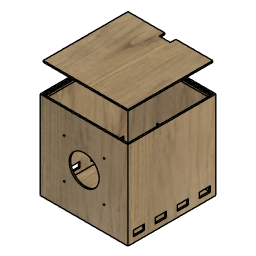
NoteBlockMaestro (Autodesk Fusion 360 design; units mm, degrees)
part number: 2025-07-01-10-41-04-519
Autodesk Fusion 360 part; units mm, degrees
sketch "Sketch1" plane through (0, 0, 0) normal (0, 0, 1) x (1, 0, 0)
  line L0 (0, 0) -> (152, 0)
  line L1 (152, 0) -> (152, -152)
  line L2 (152, -152) -> (0, -152)
  line L3 (0, -152) -> (0, 0)
  dimension "d1" = 152
  dimension "d2" = 152
  constraint horizontal L0
  constraint vertical L1
  constraint horizontal L2
  constraint vertical L3
  constraint coincident L0.start L3.end
  measures "d1" distance of L0.start L0.end
  measures "d2" distance of L0.start L2.end
extrude "Extrude1" add sketch "Sketch1" along normal blind 152 makes body 1
move_body "Move1" bodies 1 to x (1, 0, 0) y (0, 1, 0) z (0, 0, 1) at (76, 0, 0)
move_body "Move2" bodies 1 to x (1, 0, 0) y (0, 1, 0) z (0, 0, 1) at (-152, 0, 0)
move_body "Move3" bodies 1 to x (1, 0, 0) y (0, 1, 0) z (0, 0, 1) at (0, -76, 0)
move_body "Move4" bodies 1 to x (1, 0, 0) y (0, 1, 0) z (0, 0, 1) at (0, 152, 0)
shell "Shell1" thickness 2.5 removed faces 1 at (-25.3333, 25.3333, 152) on bodies 1
sketch "Sketch2" plane through (0, 0, 152) normal (0, 0, 1) x (-1, 0, 0)
  line L0 (73.5, 73.5) -> (73.5, -73.5)
  line L1 (73.5, -73.5) -> (-73.5, -73.5)
  line L2 (-73.5, -73.5) -> (-73.5, 73.5)
  line L3 (-73.5, 73.5) -> (73.5, 73.5)
  line L4 (76, 76) -> (-76, 76)
  line L5 (-76, 76) -> (-76, -76)
  line L6 (-76, -76) -> (76, -76)
  line L7 (76, -76) -> (76, 76)
  line L8 (76, -76) -> (-76, -76)
  line L9 (-76, -76) -> (-76, 76)
  line L10 (-76, 76) -> (76, 76)
  line L11 (76, 76) -> (76, -76)
  constraint horizontal L8
  constraint vertical L9
  constraint horizontal L10
  constraint vertical L11
  constraint coincident L4.end L5.start
  constraint coincident L6.end L7.start
extrude "Extrude2" add sketch "Sketch2" along normal blind 2.5 separate body contours L0 L1 L2 L3 makes body 2
move_body "Move5" bodies 2 to x (1, 0, 0) y (0, 1, 0) z (0, 0, 1) at (0, 0, 100)
ref_plane "WorkPlane1" through (0, 0, 149.5) normal (0, 0, 1) x (1, 0, 0)
sketch "Sketch3" plane through (0, 0, 149.5) normal (0, 0, 1) x (1, 0, 0)
  line L0 (73.5, 73.5) -> (-73.5, 73.5)
  line L1 (-73.5, 73.5) -> (-73.5, -73.5)
  line L2 (-73.5, -73.5) -> (73.5, -73.5)
  line L3 (73.5, -73.5) -> (73.5, 73.5)
  line L4 (-72.5, -72.5) -> (72.5, -72.5)
  line L5 (72.5, -72.5) -> (72.5, 72.5)
  line L6 (72.5, 72.5) -> (-72.5, 72.5)
  line L7 (-72.5, 72.5) -> (-72.5, -72.5)
  point P0 (-73.5, 73.5)
  point P1 (73.5, 73.5)
  point P2 (-73.5, -73.5)
  point P3 (73.5, -73.5)
  dimension "d9" = -1
  constraint horizontal L0
  constraint vertical L1
  constraint horizontal L2
  constraint vertical L3
  constraint coincident P2 L1.end
  constraint coincident P1 L0.start
extrude "Extrude3" add sketch "Sketch3" against normal blind 2 bodies 1
extrude "Extrude4" add 1 faces at (-72.5, 24.1667, 148.8333) along direction (1, 0, 0) blind 1 on bodies 1 bodies 1
extrude "Extrude5" add 1 faces at (24.5, 72.5, 148.8333) along direction (0, -1, 0) blind 1 on bodies 1 bodies 1
extrude "Extrude6" add 1 faces at (72.5, -24.5, 148.8333) along direction (-1, 0, 0) blind 1 on bodies 1 bodies 1
extrude "Extrude7" add 1 faces at (-23.8333, -72.5, 148.1667) along direction (0, 1, 0) blind 1 on bodies 1 bodies 1
extrude "Extrude8" add 1 faces at (-73.5, -24.5, 252.8333) along direction (-1, 0, 0) blind 0.1 on bodies 2 bodies 2
extrude "Extrude9" cut 1 faces at (-73.6, -24.5, 252.8333) along direction (1, 0, 0) blind 0.2 on bodies 2 bodies 2
extrude "Extrude10" cut 1 faces at (24.5333, -73.5, 252.8333) along direction (0, 1, 0) blind 0.2 on bodies 2 bodies 2
extrude "Extrude11" cut 1 faces at (73.5, 24.5667, 252.8333) along direction (-1, 0, 0) blind 0.2 on bodies 2 bodies 2
extrude "Extrude12" cut 1 faces at (-24.5, 73.5, 253.6667) along direction (0, -1, 0) blind 0.2 on bodies 2 bodies 2
move_body "Move6" bodies 2 to x (1, 0, 0) y (0, 1, 0) z (0, 0, 1) at (0, 0, -60)
sketch "Sketch4" plane through (0, 0, 194.5) normal (0, 0, 1) x (-1, 0, 0)
  line L0 (-73.3, -73.3) -> (73.4, -73.3)
  line L1 (73.4, -73.3) -> (73.4, 73.3)
  line L2 (73.4, 73.3) -> (-73.3, 73.3)
  line L3 (-73.3, 73.3) -> (-73.3, -73.3)
  line L4 (0.05, -73.3) -> (9.55, -73.3)
  line L5 (0.05, -73.3) -> (-9.45, -73.3)
  line L6 (-9.45, -73.3) -> (-9.45, -63.8)
  line L7 (-9.45, -63.8) -> (0.05, -63.8)
  line L8 (0.05, -63.8) -> (9.55, -63.8)
  line L9 (9.55, -63.8) -> (9.55, -73.3)
  dimension "d30" = 9.5
  dimension "d31" = 9.5
  dimension "d32" = 9.5
  dimension "d33" = 9.5
  dimension "d34" = 9.5
  dimension "d35" = 9.5
  constraint midpoint L0 L4.start
  constraint parallel L0 L4
  constraint parallel L0 L5
  constraint perpendicular L5 L6
  constraint perpendicular L6 L7
  constraint perpendicular L6 L8
  constraint perpendicular L4 L9
  measures "d30" distance of L4.start L4.end
  measures "d31" distance of L4.start L5.end
  measures "d32" distance of L5.end L6.end
  measures "d33" distance of L6.end L7.end
  measures "d34" distance of L7.end L8.end
  measures "d35" distance of L8.end L4.end
extrude "Extrude13" cut sketch "Sketch4" against normal blind 2.5 contours L0 L4 L5 L6 L7 L8 L9 bodies 2
move_body "Move7" bodies 2 to x (1, 0, 0) y (0, 1, 0) z (0, 0, 1) at (0, 0, -42.5)
sketch "Sketch5" plane through (0, 0, 149.5) normal (0, 0, 1) x (-1, 0, 0)
  line L0 (71.5, 71.5) -> (71.5, -71.5)
  line L1 (71.5, -71.5) -> (-71.5, -71.5)
  line L2 (-71.5, -71.5) -> (-71.5, 71.5)
  line L3 (-71.5, 71.5) -> (71.5, 71.5)
  line L4 (-73.5, 73.5) -> (-73.5, -73.5)
  line L5 (-73.5, -73.5) -> (73.5, -73.5)
  line L6 (73.5, -73.5) -> (73.5, 73.5)
  line L7 (73.5, 73.5) -> (-73.5, 73.5)
  line L8 (9.55, -73.5) -> (-9.4425, -73.5)
  line L9 (-9.4425, -73.5) -> (-9.4425, -71.5)
  line L10 (-9.4425, -71.5) -> (9.55, -71.5)
  line L11 (9.55, -71.5) -> (9.55, -73.5)
  constraint horizontal L8
  constraint vertical L9
  constraint horizontal L10
  constraint vertical L11
  constraint coincident L1 L9.end
  constraint coincident L5 L8.start
extrude "Extrude14" cut sketch "Sketch5" against normal blind 2 contours L1 L5 L8 L9 L10 L11 bodies 1
move_body "Move8" bodies 2 to x (1, 0, 0) y (0, 1, 0) z (0, 0, 1) at (0, 0, 50)
extrude "Extrude15" add 1 faces at (71.5, -23.8333, 148.1667) along direction (-1, 0, 0) blind 0.5 on bodies 1 bodies 1
extrude "Extrude16" add 1 faces at (50.4808, 71.5, 148.8333) along direction (0, -1, 0) blind 0.5 on bodies 1 bodies 1
extrude "Extrude17" add 1 faces at (-71.5, 23.8333, 148.1667) along direction (1, 0, 0) blind 0.5 on bodies 1 bodies 1
extrude "Extrude18" add 1 faces at (-23.6667, -71.5, 148.8333) along direction (0, 1, 0) blind 0.5 on bodies 1 bodies 1
extrude "Extrude19" add 1 faces at (-23.6667, -72.6667, 147.5) along direction (0, 0, -1) blind 0.5 on bodies 1 bodies 1
extrude "Extrude20" add 1 faces at (-23.6667, -72.6667, 147) along direction (0, 0, -1) blind 1 on bodies 1 bodies 1
scale "Scale1" factor 1.157895 about (71, -71, 146) bodies 1 2
move_face "MoveFace1" by (70, 0, 0) 1 faces at (-40.5439, 99.2105, 94.2807) on bodies 1
move_body "Move9" bodies 1 2 to x (1, 0, 0) y (0, 1, 0) z (0, 0, 1) at (11, 0, 0)
move_body "Move10" bodies 1 2 to x (1, 0, 0) y (0, 1, 0) z (0, 0, 1) at (0, -11, 0)
move_body "Move11" bodies 1 2 to x (1, 0, 0) y (0, 1, 0) z (0, 0, 1) at (0, 0, 23)
sketch "Sketch8" plane through (0, 88.2105, 0) normal (0, 1, 0) x (-1, 0, 0)
  line L0 (-87.7895, -0.0526) -> (88.2105, -0.0526)
  line L1 (88.2105, -0.0526) -> (88.2105, 175.9474)
  line L2 (88.2105, 175.9474) -> (-87.7895, 175.9474)
  line L3 (-87.7895, 175.9474) -> (-87.7895, -0.0526)
  line L4 (0, 25) -> (27.5, 25)
  line L5 (0, 25) -> (-27.5, 25)
  line L6 (-27.5, 25) -> (-27.5, 69)
  line L7 (-27.5, 69) -> (27.5, 69)
  line L8 (27.5, 69) -> (27.5, 25)
  dimension "d54" = 27.5
  dimension "d55" = 27.5
  dimension "d56" = 44
  dimension "d57" = 55
  constraint horizontal L4
  constraint horizontal L5
  constraint perpendicular L5 L6
  constraint perpendicular L6 L7
  measures "d54" distance of L4.start L4.end
  measures "d55" distance of L4.start L5.end
  measures "d56" distance of L5.end L6.end
  measures "d57" distance of L6.end L7.end
extrude "Extrude21" cut sketch "Sketch8" against normal blind 3 contours L4 L5 L6 L7 L8 bodies 1
sketch "Sketch9" plane through (-88.2105, 0, 0) normal (-1, 0, 0) x (0, -1, 0)
  line L0 (-88.2105, -0.0526) -> (87.7895, -0.0526)
  line L1 (87.7895, -0.0526) -> (87.7895, 175.9474)
  line L2 (87.7895, 175.9474) -> (-88.2105, 175.9474)
  line L3 (-88.2105, 175.9474) -> (-88.2105, -0.0526)
  line L4 (11, 11) -> (11, 22)
  line L5 (11, 22) -> (33, 22)
  line L6 (33, 22) -> (33, 11)
  line L7 (33, 11) -> (11, 11)
  line L8 (55, 22) -> (77, 22)
  line L9 (77, 22) -> (77, 11)
  line L10 (77, 11) -> (55, 11)
  line L11 (55, 11) -> (55, 22)
  line L12 (-11, 11) -> (-33, 11)
  line L13 (-33, 11) -> (-33, 22)
  line L14 (-33, 22) -> (-11, 22)
  line L15 (-11, 22) -> (-11, 11)
  line L16 (-55, 11) -> (-77, 11)
  line L17 (-77, 11) -> (-77, 22)
  line L18 (-77, 22) -> (-55, 22)
  line L19 (-55, 22) -> (-55, 11)
  dimension "d61" = 11
  dimension "d62" = 22
  dimension "d64" = 22
  dimension "d65" = 11
  dimension "d67" = 22
  dimension "d68" = 11
  constraint perpendicular L4 L5
  constraint perpendicular L5 L6
  constraint perpendicular L4 L7
  constraint perpendicular L0 L9
  constraint perpendicular L6 L10
  constraint perpendicular L12 L13
  constraint perpendicular L13 L14
  constraint perpendicular L13 L16
  constraint perpendicular L13 L18
  constraint perpendicular L16 L19
  measures "d61" distance of L4.start L4.end
  measures "d62" distance of L4.end L5.end
  measures "d64" distance of L8.start L8.end
  measures "d65" distance of L8.end L9.end
  measures "d67" distance of L12.start L12.end
  measures "d68" distance of L12.end L13.end
extrude "Extrude22" cut sketch "Sketch9" against normal blind 3 contours L16 L17 L18 L19 bodies 1
extrude "Extrude23" cut sketch "Sketch9" against normal blind 3 contours L12 L13 L14 L15 bodies 1
extrude "Extrude24" cut sketch "Sketch9" against normal blind 3 contours L4 L5 L6 L7 bodies 1
extrude "Extrude25" cut sketch "Sketch9" against normal blind 3 contours L8 L9 L10 L11 bodies 1
sketch "Sketch10" plane through (87.7895, 0, 0) normal (1, 0, 0) x (0, 1, 0)
  line L0 (-87.7895, -0.0526) -> (88.2105, -0.0526)
  line L1 (88.2105, -0.0526) -> (88.2105, 175.9474)
  line L2 (88.2105, 175.9474) -> (-87.7895, 175.9474)
  line L3 (-87.7895, 175.9474) -> (-87.7895, -0.0526)
  line L4 (11, 11) -> (33, 11)
  line L5 (33, 11) -> (33, 22)
  line L6 (33, 22) -> (11, 22)
  line L7 (11, 22) -> (11, 11)
  line L8 (55, 11) -> (77, 11)
  line L9 (77, 11) -> (77, 22)
  line L10 (77, 22) -> (55, 22)
  line L11 (55, 22) -> (55, 11)
  line L12 (-11, 11) -> (-33, 11)
  line L13 (-33, 11) -> (-33, 22)
  line L14 (-33, 22) -> (-11, 22)
  line L15 (-11, 22) -> (-11, 11)
  line L16 (-55, 11) -> (-77, 11)
  line L17 (-77, 11) -> (-77, 22)
  line L18 (-77, 22) -> (-55, 22)
  line L19 (-55, 22) -> (-55, 11)
  dimension "d78" = 22
  dimension "d80" = 22
  dimension "d81" = 11
  dimension "d82" = 22
  constraint perpendicular L4 L5
  constraint perpendicular L5 L6
  constraint perpendicular L5 L8
  constraint perpendicular L4 L9
  constraint perpendicular L9 L10
  constraint perpendicular L12 L13
  constraint perpendicular L13 L14
  constraint perpendicular L13 L16
  constraint perpendicular L16 L17
  constraint perpendicular L17 L18
  measures "d78" distance of L4.start L4.end
  measures "d80" distance of L12.start L12.end
  measures "d81" distance of L16.end L17.end
  measures "d82" distance of L17.end L18.end
extrude "Extrude26" cut sketch "Sketch10" against normal blind 3 contours L16 L17 L18 L19 bodies 1
extrude "Extrude27" cut sketch "Sketch10" against normal blind 3 contours L12 L13 L14 L15 bodies 1
extrude "Extrude28" cut sketch "Sketch10" against normal blind 3 contours L4 L5 L6 L7 bodies 1
extrude "Extrude29" cut sketch "Sketch10" against normal blind 3 contours L8 L9 L10 L11 bodies 1
move_face "MoveFace2" by (0, 0, -5) 1 faces at (29.1228, -87.7895, 117.2807) on bodies 1
sketch "Sketch11" plane through (0, -87.7895, 0) normal (0, -1, 0) x (1, 0, 0)
  line L0 (-88.2105, -0.0526) -> (87.7895, -0.0526)
  line L1 (87.7895, -0.0526) -> (87.7895, 175.9474)
  line L2 (87.7895, 175.9474) -> (-88.2105, 175.9474)
  line L3 (-88.2105, 175.9474) -> (-88.2105, -0.0526)
  line L4 (0, -0.0526) -> (0, 87.9474)
  circle A0 centre (0, 87.9474) radius 30
  circle A1 centre (39.8461, 128.004) radius 1.5
  circle A2 centre (39.8461, 47.8907) radius 1.5
  circle A3 centre (-40.0567, 48.1012) radius 1.5
  circle A4 centre (-40.0567, 127.7935) radius 1.5
  dimension "d91" = 88
  dimension "d92" = 60
  dimension "d94" = 3
  dimension "d95" = 3
  dimension "d96" = 3
  dimension "d97" = 3
  constraint coincident L4.end A0.centre
  measures "d91" distance of L4.start L4.end
  measures "d92" diameter of A0
  measures "d94" diameter of A1
  measures "d95" diameter of A2
  measures "d96" diameter of A3
  measures "d97" diameter of A4
extrude "Extrude30" cut sketch "Sketch11" against normal blind 3 contours A1 bodies 1
extrude "Extrude31" cut sketch "Sketch11" against normal blind 3 contours A0 bodies 1
extrude "Extrude32" cut sketch "Sketch11" against normal blind 3 contours A4 bodies 1
extrude "Extrude33" cut sketch "Sketch11" against normal blind 3 contours A3 bodies 1
extrude "Extrude34" cut sketch "Sketch11" against normal blind 3 contours A2 bodies 1
equation "d52 = 22 / 19"
